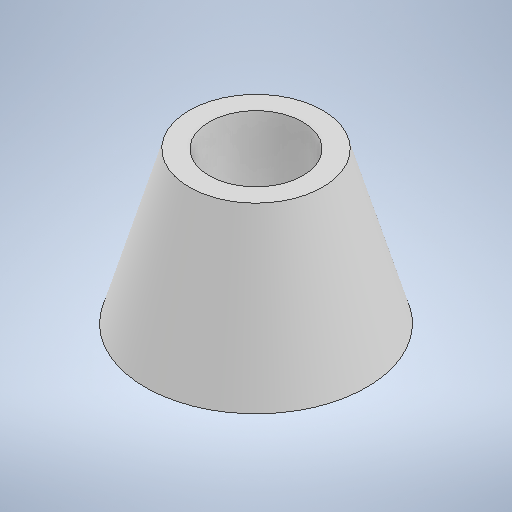
# Autodesk Inventor part: Energy Absorption Crush
Saved by Autodesk Inventor 2026.2 (Build 302298000, 298)
## iProperties
Created: 2026-01-18
Part Number: Energy Absorption Crush
Material: Generic
Document SubType Name: Modeling
Designer: daryu
Density: 1 g/cm^3
Appearance: Default
Author: daryu
Autodesk Inventor part; units mm, degrees
ref_plane "YZ Plane" through (0, 0, 0) normal (1, 0, 0) x (0, 1, 0)
ref_plane "XZ Plane" through (0, 0, 0) normal (0, 1, 0) x (-1, 0, 0)
ref_plane "XY Plane" through (0, 0, 0) normal (0, 0, 1) x (1, 0, 0)
sketch "Sketch1" plane through (0, 0, 0) normal (0, 0, 1) x (1, 0, 0)
  arc A0 (-29.9776, 14.7762) -> (0, 0) centre (9.8435, 57.7672) ccw
  line L0 (-14.7987, 4.6004) -> (-8.912, 24.8392)
  line L1 (0, 24.8392) -> (-8.912, 24.8392)
  line L2 (0, 0) -> (0, 24.8392)
  dimension "d0" = 21.0774
  dimension "d1" = 8.912
  dimension "d2" = 24.8392
  dimension "d3" = 58.5999
  constraints: 6 end point, 3 point on circle, 1 centre point, 1 coincident
  measures "d0" distance of L0.start L0.end
  measures "d1" distance of L1.start L0.end
  measures "d2" distance of L2.start L1.start
  measures "d3" radius of A0
revolve "Revolution1" add sketch "Sketch1" angle 360 about axis through (0, 0, 0) along (0, 1, 0)
sketch "Sketch2" plane through (0, 24.8392, 0) normal (0, 1, 0) x (1, 0, 0)
  circle A0 centre (0, 0) radius 6.25
  dimension "d5" = 12.5
  constraints: 1 centre point, 1 coincident
  measures "d5" diameter of A0
hole "Hole1" at (0, 24.8392, 0) direction (0, -1, 0) diameter 12.5 depth 9
body "Solid1"
